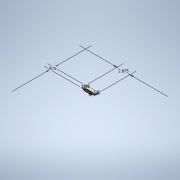
# Autodesk Inventor part: Compute Module Top Cover for RoadBot Rail-r1
Saved by Autodesk Inventor 2020 (Build 240168000, 168)
## iProperties
Created: 2022-03-31
Part Number: Compute Module Top Cover for RoadBot Rail-r1
Material: Generic
Document SubType Name: Modeling
Designer: Beaucage
Density: 1 g/cm^3
Appearance: Default
Author: Beaucage
Autodesk Inventor part; units mm, degrees
ref_plane "YZ Plane" through (0, 0, 0) normal (1, 0, 0) x (0, 1, 0)
ref_plane "XZ Plane" through (0, 0, 0) normal (0, 1, 0) x (-1, 0, 0)
ref_plane "XY Plane" through (0, 0, 0) normal (0, 0, 1) x (1, 0, 0)
sketch "Sketch1" plane through (0, 0, 0) normal (0, 1, 0) x (-1, 0, 0)
  line L0 (0, 0) -> (73.025, 0)
  line L1 (73.025, 0) -> (73.025, -22.225)
  line L2 (73.025, -22.225) -> (0, -22.225)
  line L3 (0, -22.225) -> (0, 0)
  line L4 (73.025, 0) -> (53.975, 0)
  line L5 (0, 0) -> (19.05, 0)
  line L6 (53.975, 0) -> (19.05, 0) construction
  line L7 (53.975, 6.35) -> (19.05, 6.35)
  line L8 (19.05, -6.35) -> (53.975, -6.35)
  arc A0 (53.975, -6.35) -> (53.975, 6.35) centre (53.975, 0) ccw
  arc A1 (19.05, 6.35) -> (19.05, -6.35) centre (19.05, 0) ccw
  line L9 (73.025, -22.225) -> (69.85, -22.225)
  line L10 (69.85, -22.225) -> (69.85, -19.05)
  line L11 (69.85, -19.05) -> (73.025, -19.05)
  line L12 (73.025, -19.05) -> (73.025, -22.225)
  line L13 (0, -22.225) -> (3.175, -22.225)
  line L14 (3.175, -22.225) -> (3.175, -19.05)
  line L15 (3.175, -19.05) -> (0, -19.05)
  line L16 (0, -19.05) -> (0, -22.225)
  point P0 (36.5125, 0)
  point P1 (60.325, 0)
  point P2 (12.7, 0)
  dimension "d0" = 73.025
  dimension "d1" = 22.225
  dimension "d2" = 19.05
  dimension "d3" = 19.05
  dimension "d4" = 12.7
  dimension "d7" = 3.175
  dimension "d8" = 3.175
  dimension "d9" = 3.175
  dimension "d10" = 3.175
  constraints: 36 end point, 7 parallel, 4 horizontal, 4 point on circle, 4 tangent, 3 perpendicular, 2 centre point, 2 point on line, 1 midpoint
  measures "d0" distance of L1.end L2.end
  measures "d1" distance of L0.end L1.end
  measures "d2" distance of L0.end L4.end
  measures "d3" distance of L0.start L5.end
  measures "d4" diameter of A1
  measures "d7" distance of L10.end L11.end
  measures "d8" distance of L9.end L10.end
  measures "d9" distance of L15.end L14.end
  measures "d10" distance of L14.end L13.end
extrude "Extrusion1" add sketch "Sketch1" along normal blind 3.175 contours A1 L8 A0 L0 L1 L11 L10 L2 L14 L15 L3 | L15 L14 L2 L3 | L1 L2 L10 L11
hole "Hole1" at (-69.85, 0, -19.05) at (-3.175, 0, -19.05) direction (0, 1, 0) diameter 3.2766 end through all counterbore diameter 5.5626 counterbore depth 1.5875 clearance for "Socket Head Cap Screw" size "#4" standard "Ansi Unified Screw Threads"
fillet "Fillet2" radius 3.175 3 edges at (-14.5599, 0, -4.4901) (-58.4651, 0, -4.4901) (-36.5125, 0, -6.35)
body "Solid1"
